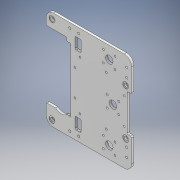
# Autodesk Inventor part: new_torso_topplate
Saved by Autodesk Inventor 2018 (Build 220112000, 112)
## iProperties
Created: 2017-02-16
Part Number: new_torso_topplate
Material: Aluminum 2014-T4
Document SubType Name: Modeling
Designer: steve
Mass: 92.2166 g
Surface Area: 250.436 cm^2
Volume: 32.9345 cm^3
Density: 2.8 g/cm^3
Appearance: Satin
torso_topplate_W: 133,000 mm
torso_topplate_l_to_fit: 82,000 mm
torso_topplate_d: 3,000 mm
fit_w: 85,000 mm
fit_d: 25,500 mm
torso_topplate_total_l: 110,000 mm
stock_6_width: 6,250 mm
pillar_block_length: 20,000 mm
pillar_block_width: 20,000 mm
pillar_width: 15,000 mm
stock_3_width: 3,000 mm
pillar_length: 80,000 mm
pillar_plate_length: 60,000 mm
cover_d: 3,500 mm
Author: steve
Autodesk Inventor part; units mm, degrees
ref_plane "YZ Plane" through (0, 0, 0) normal (1, 0, 0) x (0, 1, 0)
ref_plane "XZ Plane" through (0, 0, 0) normal (0, 1, 0) x (-1, 0, 0)
ref_plane "XY Plane" through (0, 0, 0) normal (0, 0, 1) x (1, 0, 0)
sketch "Sketch1" plane through (0, 0, 0) normal (0, 1, 0) x (-1, 0, 0)
  line L0 (-41, 66.5) -> (41, 66.5) construction
  line L1 (41, 66.5) -> (41, -66.5) construction
  line L2 (41, -66.5) -> (-41, -66.5) construction
  line L3 (-41, -66.5) -> (-41, 66.5) construction
  line L4 (-41, 66.5) -> (41, -66.5) construction
  line L5 (41, 66.5) -> (-41, -66.5) construction
  line L6 (106.5296, 0) -> (-65.5883, 0) construction
  line L7 (66.5, -42.5) -> (61.25, -42.5) construction
  line L8 (41, -42.5) -> (41, 42.5) construction
  line L9 (41, 42.5) -> (66.5, 42.5) construction
  line L10 (66.5, 42.5) -> (66.5, -42.5) construction
  line L11 (66.5, -42.5) -> (41, 42.5) construction
  line L12 (41, -42.5) -> (66.5, 42.5) construction
  line L13 (74, 66.5) -> (74, -66.5) construction
  line L14 (-41, 66.5) -> (74, 66.5)
  line L15 (74, 66.5) -> (74, -66.5)
  line L16 (74, -66.5) -> (-41, -66.5)
  line L17 (-41, -66.5) -> (-41, 66.5)
  circle A0 centre (65.4393, 41.4393) radius 1.5 construction
  line L18 (66.5, 42.5) -> (60.0868, 36.0868) construction
  line L19 (66.5, 42.5) -> (75.5696, 42.5) construction
  line L20 (66.5, -42.5) -> (64.7221, -40.7221) construction
  line L21 (66.5, -42.5) -> (69.0143, -42.5) construction
  line L22 (41, -42.5) -> (42.6048, -40.8952) construction
  line L23 (41, -42.5) -> (43.2695, -42.5) construction
  line L24 (41, 42.5) -> (46.0799, 37.4201) construction
  line L25 (41, 42.5) -> (48.184, 42.5) construction
  circle A1 centre (42.0607, 41.4393) radius 1.5 construction
  circle A2 centre (65.4393, -41.4393) radius 1.5 construction
  circle A3 centre (42.0607, -41.4393) radius 1.5 construction
  line L26 (43.1213, 42.5) -> (46.25, 42.5)
  line L27 (66.5, 40.3787) -> (66.5, -40.3787)
  line L28 (64.3787, -42.5) -> (61.25, -42.5)
  line L29 (41, -40.3787) -> (41, 40.3787)
  arc A4 (66.5, 40.3787) -> (64.3787, 42.5) centre (65.4393, 41.4393) ccw construction
  arc A5 (64.3787, -42.5) -> (66.5, -40.3787) centre (65.4393, -41.4393) ccw construction
  arc A6 (41, -40.3787) -> (43.1213, -42.5) centre (42.0607, -41.4393) ccw
  arc A7 (43.1213, 42.5) -> (41, 40.3787) centre (42.0607, 41.4393) ccw
  line L30 (81.9414, -45.5) -> (23.4915, -45.5) construction
  line L31 (53.75, 61.7827) -> (53.75, -107.6212) construction
  line L32 (46.25, -34.6173) -> (61.25, -34.6173) construction
  line L33 (61.25, -34.6173) -> (61.25, -50.3827) construction
  line L34 (61.25, -50.3827) -> (46.25, -50.3827) construction
  line L35 (46.25, -50.3827) -> (46.25, -34.6173) construction
  line L36 (46.25, -34.6173) -> (61.25, -50.3827) construction
  line L37 (61.25, -34.6173) -> (46.25, -50.3827) construction
  arc A8 (46.25, -42.5) -> (61.25, -42.5) centre (53.75, -34.625) ccw
  line L38 (61.25, -42.5) -> (41, -42.5) construction
  line L39 (61.25, -42.5) -> (46.25, -42.5) construction
  line L40 (46.25, -42.5) -> (43.1213, -42.5)
  arc A9 (61.25, 42.5) -> (46.25, 42.5) centre (53.75, 34.625) ccw
  line L41 (61.25, 42.5) -> (64.3787, 42.5)
  line L42 (46.25, 42.5) -> (61.25, 42.5) construction
  line L43 (64.3787, 42.5) -> (66.5, 42.5)
  line L44 (66.5, 42.5) -> (66.5, 40.3787)
  line L45 (64.3787, -42.5) -> (66.5, -42.5)
  line L46 (66.5, -42.5) -> (66.5, -40.3787)
  point P0 (0, 0)
  point P1 (53.75, 0)
  point P2 (53.75, 0)
  point P3 (53.75, -42.5)
  dimension "d0" = 133
  dimension "d1" = 82
  dimension "d2" = 25.5
  dimension "d3" = 85
  dimension "d4" = 7.5
  dimension "d6" = 3
  dimension "d7" = 135
  dimension "d8" = 135
  dimension "d9" = 45
  dimension "d10" = 45
  dimension "d11" = 3
  dimension "d12" = 3
  dimension "d13" = 3
  dimension "d99" = 15
  dimension "d100" = 3
  constraints: 92 end point, 24 point on circle, 17 point on line, 11 horizontal, 11 midpoint, 10 centre point, 9 parallel, 5 perpendicular, 4 coincident, 4 equal length, 3 collinear, 3 symmetric about line, 2 vertical, 1 tangent, 1 other
  measures "d0" distance of L0.end L1.end
  measures "d1" distance of L1.end L2.end
  measures "d2" distance of L7.start L8.start
  measures "d3" distance of L9.end L7.start
  measures "d4" distance between parallel lines of L13 L10
  measures "d6" diameter of A0
  measures "d7" angle of L18 L19
  measures "d8" angle of L21 L20
  measures "d9" angle of L23 L22
  measures "d10" angle of L24 L25
  measures "d11" diameter of A3
  measures "d12" diameter of A2
  measures "d13" diameter of A1
  measures "d99" distance of L33.end L34.end
  measures "d100" distance between parallel lines of L7 L30
extrude "Extrusion1" add sketch "Sketch1" along normal blind 3
fillet "Fillet1" radius 10 4 edges at (41, 1.5, 66.5) (41, 1.5, -66.5) (-74, 1.5, -66.5) (-74, 1.5, 66.5)
sketch "Sketch2" plane through (0, 3, 0) normal (0, 1, 0) x (1, 0, 0)
  arc A0 (-74, -56.5) -> (-64, -66.5) centre (-64, -56.5) ccw construction
  line L0 (-64, -66.5) -> (31, -66.5) construction
  arc A1 (31, -66.5) -> (41, -56.5) centre (31, -56.5) ccw construction
  line L1 (41, -56.5) -> (41, 56.5) construction
  arc A2 (41, 56.5) -> (31, 66.5) centre (31, 56.5) ccw construction
  line L2 (31, 66.5) -> (-64, 66.5) construction
  arc A3 (-64, 66.5) -> (-74, 56.5) centre (-64, 56.5) ccw construction
  line L3 (-74, 56.5) -> (-74, -56.5) construction
  line L4 (-66.5, -42.5) -> (-66.5, 42.5) construction
  line L5 (-66.5, 42.5) -> (-61.25, 42.5) construction
  arc A4 (-41, 40.3787) -> (-43.1213, 42.5) centre (-42.0607, 41.4393) ccw construction
  line L6 (-41, 40.3787) -> (-41, -40.3787) construction
  arc A5 (-43.1213, -42.5) -> (-41, -40.3787) centre (-42.0607, -41.4393) ccw construction
  line L7 (-43.1213, -42.5) -> (-46.25, -42.5) construction
  line L8 (31.25, -56.5) -> (37.5, -56.5) construction
  line L9 (37.5, -56.5) -> (37.5, -36.5) construction
  line L10 (37.5, -36.5) -> (31.25, -36.5) construction
  line L11 (31.25, -36.5) -> (31.25, -56.5) construction
  line L12 (37.5, 78) -> (37.5, -82) construction
  line L13 (41, -56.5) -> (-13.5, -56.5) construction
  line L14 (41, -56.5) -> (41, 56.5) construction
  line L15 (41, 56.5) -> (10.5, 56.5) construction
  line L16 (31.25, 36.5) -> (37.5, 36.5) construction
  line L17 (37.5, 36.5) -> (37.5, 56.5) construction
  line L18 (37.5, 56.5) -> (31.25, 56.5) construction
  line L19 (31.25, 56.5) -> (31.25, 36.5) construction
  line L20 (34.375, -36.5) -> (34.375, -56.5) construction
  line L21 (34.375, 36.5) -> (34.375, 56.5) construction
  line L22 (31.25, 46.5) -> (48, 46.5) construction
  line L23 (31.25, -46.5) -> (52, -46.5) construction
  line L24 (-75, -63) -> (42, -63) construction
  line L25 (-71, 63) -> (42, 63) construction
  line L26 (-46, -105.44) -> (-46, 104.2053) construction
  line L27 (-41, 40.3787) -> (-41, -40.3787) construction
  line L28 (-46, -63) -> (-26, -63) construction
  line L29 (-26, -63) -> (-26, -56.75) construction
  line L30 (-26, -56.75) -> (-46, -56.75) construction
  line L31 (-46, -56.75) -> (-46, -63) construction
  line L32 (-46, -59.875) -> (-26, -59.875) construction
  line L33 (-36, -56.75) -> (-36, -63) construction
  line L34 (-46, 56.75) -> (-26, 56.75) construction
  line L35 (-26, 56.75) -> (-26, 63) construction
  line L36 (-26, 63) -> (-46, 63) construction
  line L37 (-46, 63) -> (-46, 56.75) construction
  line L38 (-46, 59.875) -> (-26, 59.875) construction
  line L39 (-36, 63) -> (-36, 56.75) construction
  arc A6 (-61.25, -42.5) -> (-46.25, -42.5) centre (-53.75, -34.625) ccw projected
  line L40 (-61.25, -42.5) -> (-66.5, -42.5) projected
  arc A7 (-46.25, 42.5) -> (-61.25, 42.5) centre (-53.75, 34.625) ccw projected
  line L41 (-46.25, 42.5) -> (-43.1213, 42.5) projected
  point P0 (0, 0)
  point P1 (34.375, -52.5)
  point P2 (34.375, -40.5)
  point P3 (34.375, 40.5)
  point P4 (34.375, 52.5)
  point P5 (-30, 59.875)
  point P6 (-42, 59.875)
  point P7 (-30, -59.875)
  point P8 (-42, -59.875)
  dimension "d17" = 20
  dimension "d18" = 6.25
  dimension "d19" = 3.5
  dimension "d20" = 20
  dimension "d21" = 6.25
  dimension "d24" = 3.5
  dimension "d25" = 3.5
  dimension "d26" = 6.25
  dimension "d27" = 20
  dimension "d28" = 6.25
  dimension "d29" = 20
  dimension "d32" = 6
  dimension "d33" = 6
  dimension "d34" = 6
  dimension "d35" = 6
  dimension "d36" = 6
  dimension "d37" = 6
  dimension "d38" = 6
  dimension "d39" = 6
  dimension "d61" = 5
  constraints: 60 end point, 13 midpoint, 10 horizontal, 9 point on line, 8 collinear, 8 parallel, 5 perpendicular, 1 vertical
  measures "d17" distance of L10.end L8.start
  measures "d18" distance of L8.start L8.end
  measures "d19" distance between parallel lines of L1 L12
  measures "d20" distance of L18.end L19.end
  measures "d21" distance of L19.end L16.end
  measures "d24" distance between parallel lines of L0 L24
  measures "d25" distance between parallel lines of L2 L25
  measures "d26" distance of L28.end L29.end
  measures "d27" distance of L29.end L30.end
  measures "d28" distance of L34.end L36.start
  measures "d29" distance of L36.start L37.start
  measures "d32" distance from line of L33 point (-42, -59.875)
  measures "d33" distance from line of L33 point (-30, -59.875)
  measures "d34" distance from line of L23 point (34.375, -52.5)
  measures "d35" distance from line of L23 point (34.375, -40.5)
  measures "d36" distance from line of L22 point (34.375, 40.5)
  measures "d37" distance from line of L22 point (34.375, 52.5)
  measures "d38" distance from line of L39 point (-30, 59.875)
  measures "d39" distance from line of L39 point (-42, 59.875)
  measures "d61" distance between parallel lines of L27 L26
hole "Hole1" at (34.375, 3, 52.5) at (34.375, 3, 40.5) at (34.375, 3, -40.5) at (34.375, 3, -52.5) at (-30, 3, -59.875) at (-42, 3, -59.875) at (-30, 3, 59.875) at (-42, 3, 59.875) direction (0, -1, 0) diameter 3 end through all countersink diameter 4 countersink angle 90
sketch "Sketch4" plane through (0, 3, 0) normal (0, 1, 0) x (1, 0, 0)
  line L0 (11, -83) -> (11, 74) construction
  line L1 (41, -56.5) -> (41, 56.5) construction
  line L2 (-83, -50) -> (80, -50) construction
  line L3 (-64, -66.5) -> (31, -66.5) construction
  circle A0 centre (11, -50) radius 5
  line L4 (112.6, 0) -> (-115.6, 0) construction
  circle A1 centre (11, 50) radius 5
  point P0 (0, 0)
  dimension "d48" = 30
  dimension "d49" = 16.5
  dimension "d50" = 10
  constraints: 4 end point, 2 centre point, 2 point on line, 1 horizontal, 1 symmetric about line, 1 vertical, 1 other
  measures "d48" distance between parallel lines of L1 L0
  measures "d49" distance between parallel lines of L2 L3
  measures "d50" diameter of A0
extrude "Extrusion2" cut sketch "Sketch4" against normal blind 3
sketch "Sketch5" plane through (0, 3, 0) normal (0, 1, 0) x (1, 0, 0)
  circle A0 centre (11, -50) radius 11 construction
  circle A1 centre (11, -50) radius 5 construction
  line L0 (18.7782, -42.2218) -> (3.2218, -42.2218) construction
  line L1 (3.2218, -42.2218) -> (3.2218, -57.7782) construction
  line L2 (3.2218, -57.7782) -> (18.7782, -57.7782) construction
  line L3 (18.7782, -57.7782) -> (18.7782, -42.2218) construction
  line L4 (18.7782, -42.2218) -> (3.2218, -57.7782) construction
  line L5 (3.2218, -42.2218) -> (18.7782, -57.7782) construction
  line L6 (-97, 0) -> (64, 0) construction
  circle A2 centre (11, 50) radius 11 construction
  circle A3 centre (11, 50) radius 5 construction
  line L7 (18.7782, 42.2218) -> (3.2218, 42.2218) construction
  line L8 (3.2218, 42.2218) -> (3.2218, 57.7782) construction
  line L9 (3.2218, 57.7782) -> (18.7782, 57.7782) construction
  line L10 (18.7782, 57.7782) -> (18.7782, 42.2218) construction
  line L11 (18.7782, 42.2218) -> (3.2218, 57.7782) construction
  line L12 (3.2218, 42.2218) -> (18.7782, 57.7782) construction
  point P0 (0, 0)
  dimension "d53" = 22
  constraints: 24 end point, 10 symmetric about line, 8 coincident, 4 midpoint, 2 horizontal, 2 parallel, 2 perpendicular, 1 centre point, 8 other
hole "Hole2" at (3.2218, 3, 42.2218) at (18.7782, 3, 42.2218) at (18.7782, 3, 57.7782) at (3.2218, 3, 57.7782) at (3.2218, 3, -57.7782) at (18.7782, 3, -57.7782) at (18.7782, 3, -42.2218) at (3.2218, 3, -42.2218) direction (0, -1, 0) diameter 2.5 end through all
sketch "Sketch6" plane through (0, 3, 0) normal (0, 1, 0) x (1, 0, 0)
  line L0 (-97, 0) -> (64, 0) construction
  circle A0 centre (16, 0) radius 5
  circle A1 centre (16, 0) radius 11 construction
  line L1 (23.7782, 7.7782) -> (8.2218, 7.7782) construction
  line L2 (8.2218, 7.7782) -> (8.2218, -7.7782) construction
  line L3 (8.2218, -7.7782) -> (23.7782, -7.7782) construction
  line L4 (23.7782, -7.7782) -> (23.7782, 7.7782) construction
  line L5 (23.7782, 7.7782) -> (8.2218, -7.7782) construction
  line L6 (8.2218, 7.7782) -> (23.7782, -7.7782) construction
  circle A2 centre (8.2218, -7.7782) radius 1.25
  circle A3 centre (8.2218, 7.7782) radius 1.25
  circle A4 centre (23.7782, -7.7782) radius 1.25
  circle A5 centre (23.7782, 7.7782) radius 1.25
  line L7 (41, -56.5) -> (41, 56.5) projected
  point P0 (0, 0)
  dimension "d63" = 22
  dimension "d62" = 10
  dimension "d64" = 2.5
  dimension "d65" = 25
  constraints: 12 end point, 5 centre point, 4 coincident, 3 equal radius, 2 midpoint, 2 parallel, 2 perpendicular, 1 horizontal, 1 point on line, 4 other
  measures "d62" diameter of A0
  measures "d64" diameter of A2
  measures "d65" distance from line of L7 A0.centre
extrude "Extrusion3" cut sketch "Sketch6" against normal through all
sketch "Sketch7" plane through (0, 0, 0) normal (0, -1, 0) x (1, 0, 0)
  line L0 (41, 56.5) -> (41, -56.5) construction
  line L1 (41, 0) -> (-82.9368, 0) construction
  line L2 (35, -25) -> (41, -25)
  line L3 (41, -25) -> (41, 25)
  line L4 (41, 25) -> (35, 25)
  line L5 (35, 25) -> (35, -25)
  line L6 (35, -25) -> (41, 25) construction
  line L7 (41, -25) -> (35, 25) construction
  point P0 (0, 0)
  point P1 (38, 0)
  dimension "d68" = 6
  dimension "d69" = 50
  constraints: 14 end point, 3 midpoint, 2 horizontal, 2 parallel, 2 point on line, 1 perpendicular
  measures "d68" distance of L2.start L2.end
  measures "d69" distance of L4.end L2.start
extrude "Extrusion4" cut sketch "Sketch7" against normal through all
fillet "Fillet2" radius 1.5 4 edges at (35, 1.5, 25) (35, 1.5, -25) (41, 1.5, -25) (41, 1.5, 25)
sketch "Sketch8" plane through (0, 3, 0) normal (0, 1, 0) x (1, 0, 0)
  line L0 (31, -17.75) -> (-35, -17.75) construction
  line L1 (-35, -17.75) -> (-35, 17.75) construction
  line L2 (-35, 17.75) -> (31, 17.75) construction
  line L3 (31, 17.75) -> (31, -17.75) construction
  line L4 (31, -17.75) -> (-35, 17.75) construction
  line L5 (-35, -17.75) -> (31, 17.75) construction
  line L6 (64, 0) -> (-97, 0) construction
  line L7 (7.0558, -33) -> (-28.4442, -33) construction
  line L8 (-28.4442, -33) -> (-28.4442, 33) construction
  line L9 (-28.4442, 33) -> (7.0558, 33) construction
  line L10 (7.0558, 33) -> (7.0558, -33) construction
  line L11 (7.0558, -33) -> (-28.4442, 33) construction
  line L12 (-28.4442, -33) -> (7.0558, 33) construction
  line L13 (-41, 40.3787) -> (-41, -40.3787) projected
  point P0 (0, 0)
  point P1 (-2, 0)
  point P2 (-2, 0)
  point P3 (-10.6942, 0)
  dimension "d73" = 35.5
  dimension "d74" = 66
  dimension "d77" = 35.5
  dimension "d78" = 66
  dimension "d115" = 6
  constraints: 24 end point, 8 coincident, 5 midpoint, 4 parallel, 2 horizontal, 2 perpendicular, 2 point on line
  measures "d73" distance of L0.end L1.end
  measures "d74" distance of L1.end L2.end
  measures "d77" distance of L8.end L9.end
  measures "d78" distance of L7.end L8.end
  measures "d115" distance between parallel lines of L1 L13
hole "Hole3" at (-28.4442, 3, 33) at (7.0558, 3, 33) at (7.0558, 3, -33) at (-28.4442, 3, -33) at (-35, 3, -17.75) at (-35, 3, 17.75) at (31, 3, 17.75) at (31, 3, -17.75) direction (0, -1, 0) diameter 2.5 end through all
sketch "Sketch10" plane through (0, 0, 0) normal (0, -1, 0) x (1, 0, 0)
  line L0 (-81.0677, 46.5) -> (54.948, 46.5) construction
  line L1 (-31, 73.2043) -> (-31, -77.9028) construction
  line L2 (31, 66.5) -> (-64, 66.5) construction
  line L3 (-108.2708, 0) -> (82.1512, 0) construction
  line L4 (-41, 40.3787) -> (-41, -40.3787) projected
  line L5 (-28.5, 38.75) -> (-33.5, 38.75)
  line L6 (-35, 40.25) -> (-35, 52.75)
  line L7 (-33.5, 54.25) -> (-28.5, 54.25)
  line L8 (-27, 52.75) -> (-27, 40.25)
  line L9 (-27, 38.75) -> (-35, 54.25) construction
  line L10 (-35, 38.75) -> (-27, 54.25) construction
  arc A0 (-35, 40.25) -> (-33.5, 38.75) centre (-33.5, 40.25) ccw
  arc A1 (-33.5, 54.25) -> (-35, 52.75) centre (-33.5, 52.75) ccw
  arc A2 (-27, 52.75) -> (-28.5, 54.25) centre (-28.5, 52.75) ccw
  arc A3 (-28.5, 38.75) -> (-27, 40.25) centre (-28.5, 40.25) ccw
  line L11 (-28.5, -38.75) -> (-33.5, -38.75)
  line L12 (-35, -40.25) -> (-35, -52.75)
  line L13 (-33.5, -54.25) -> (-28.5, -54.25)
  line L14 (-27, -52.75) -> (-27, -40.25)
  arc A4 (-33.5, -38.75) -> (-35, -40.25) centre (-33.5, -40.25) ccw
  arc A5 (-35, -52.75) -> (-33.5, -54.25) centre (-33.5, -52.75) ccw
  arc A6 (-28.5, -54.25) -> (-27, -52.75) centre (-28.5, -52.75) ccw
  arc A7 (-27, -40.25) -> (-28.5, -38.75) centre (-28.5, -40.25) ccw
  point P0 (0, 0)
  point P1 (-31, 46.5)
  dimension "d92" = 20
  dimension "d95" = 10
  dimension "d96" = 15.5
  dimension "d97" = 8
  dimension "d98" = 1.5
  constraints: 24 end point, 16 point on circle, 12 symmetric about line, 10 point on line, 8 centre point, 8 tangent, 3 equal radius, 2 horizontal, 2 midpoint, 2 parallel, 1 perpendicular, 1 vertical, 4 other
  measures "d92" distance between parallel lines of L2 L0
  measures "d95" distance between parallel lines of L4 L1
  measures "d96" distance of L10.start L9.end
  measures "d97" distance of L9.end L10.end
  measures "d98" radius of A0
extrude "Extrusion6" cut sketch "Sketch10" against normal through all
sketch "Sketch11" plane through (0, 3, 0) normal (0, 1, 0) x (1, 0, 0)
  line L0 (38, -57.2977) -> (38, -10.4213) construction
  circle A0 centre (33, -31) radius 5 construction
  line L1 (35, -23.5) -> (35, 23.5) construction
  line L2 (-97, 0) -> (64, 0) construction
  line L3 (39.5, -25) -> (36.5, -25) construction
  line L4 (41, -56.5) -> (41, -26.5) construction
  circle A1 centre (-66, -58.5) radius 5 construction
  line L5 (-71, -65.8975) -> (-71, -94.3992) construction
  line L6 (-74, 56.5) -> (-74, -56.5) construction
  line L7 (-64, -66.5) -> (31, -66.5) construction
  circle A2 centre (33, 31) radius 5 construction
  circle A3 centre (-66, 58.5) radius 5 construction
  point P0 (0, 0)
  dimension "d101" = 10
  dimension "d103" = 6
  dimension "d104" = 3
  dimension "d105" = 10
  dimension "d106" = 3
  dimension "d107" = 8
  constraints: 4 centre point, 4 end point, 3 coincident, 3 symmetric about line, 2 tangent, 2 vertical, 2 other
  measures "d101" diameter of A0
  measures "d103" distance from line of L3 A0.centre
  measures "d104" distance between parallel lines of L0 L4
  measures "d105" diameter of A1
  measures "d106" distance between parallel lines of L6 L5
  measures "d107" distance from line of L7 A1.centre
hole "Hole4" at (-66, 3, 58.5) at (33, 3, 31) at (-66, 3, -58.5) at (33, 3, -31) direction (0, -1, 0) diameter 5 end through all
sketch "Sketch13" plane through (0, 3, 0) normal (0, 1, 0) x (1, 0, 0)
  line L0 (-74, -56.5) -> (-74, 56.5) projected
  line L1 (-66.5, -42.5) -> (-74, -42.5)
  line L2 (-74, -42.5) -> (-74, 42.5)
  line L3 (-74, 42.5) -> (-66.5, 42.5)
  line L4 (-66.5, 42.5) -> (-66.5, -42.5)
  line L5 (-66.5, 42.5) -> (-61.25, 42.5) projected
  point P0 (0, 0)
  constraints: 8 end point, 2 parallel, 1 collinear, 1 horizontal, 1 perpendicular, 1 point on line
extrude "Extrusion7" cut sketch "Sketch13" against normal through all
fillet "Fillet4" radius 1.5 2 edges at (-74, 1.5, 42.5) (-74, 1.5, -42.5)
sketch "Sketch14" plane through (0, 0, 0) normal (0, -1, 0) x (1, 0, 0)
  circle A0 centre (33, 31) radius 2.5 projected
  circle A1 centre (-66, 58.5) radius 2.5 projected
  circle A2 centre (-66, -58.5) radius 2.5 projected
  circle A3 centre (33, -31) radius 2.5 projected
  circle A4 centre (33, 31) radius 4.05
  circle A5 centre (-66, 58.5) radius 4.05
  circle A6 centre (33, -31) radius 4.05
  circle A7 centre (-66, -58.5) radius 4.05
  point P0 (0, 0)
  dimension "d119" = 8.1
  dimension "d120" = 8.1
  dimension "d121" = 8.1
  dimension "d122" = 8.1
  constraints: 4 centre point, 4 coincident
  measures "d119" diameter of A4
  measures "d120" diameter of A6
  measures "d121" diameter of A5
  measures "d122" diameter of A7
extrude "Extrusion8" cut sketch "Sketch14" against normal blind 0.5
sketch "Sketch15" plane through (0, 0, 0) normal (0, -1, 0) x (1, 0, 0)
  line L0 (-46.25, 42.5) -> (-74, 42.5)
  line L1 (-74, 42.5) -> (-74, 47.5)
  line L2 (-74, 47.5) -> (-46.25, 47.5)
  line L3 (-46.25, 47.5) -> (-46.25, 42.5)
  line L4 (-74, 56.5) -> (-74, 44) projected
  point P0 (0, 0)
  dimension "d129" = 5
  constraints: 8 end point, 2 parallel, 1 coincident, 1 collinear, 1 horizontal, 1 perpendicular
  measures "d129" distance of L2.end L0.start
extrude "Extrusion9" cut sketch "Sketch15" against normal through all
fillet "Fillet6" radius 1.5 3 edges at (-46.25, 1.5, 42.5) (-46.25, 1.5, 47.5) (-74, 1.5, 47.5)
fillet_without_effect "Fillet7"
equation "\"d0\" = torso_topplate_W"
equation "\"d1\" = torso_topplate_l_to_fit"
equation "\"d2\" = fit_d"
equation "\"d3\" = fit_w"
equation "\"d14\" = torso_topplate_d"
equation "\"d17\" = pillar_block_width"
equation "\"d18\" = stock_6_width"
equation "\"d19\" = cover_d"
equation "\"d20\" = d22"
equation "\"d21\" = d23"
equation "\"d24\" = cover_d"
equation "\"d25\" = cover_d"
equation "\"d26\" = stock_6_width"
equation "\"d27\" = pillar_block_width"
equation "\"d28\" = d30"
equation "\"d29\" = d31"
equation "\"d61\" = back_pillar_to_fit"
equation "\"d51\" = torso_topplate_d"
equation "\"d65\" = head_fix_dist"
equation "\"torso_topplate_W\" = 133"
equation "\"torso_topplate_l_to_fit\" = 82"
equation "\"torso_topplate_d\" = 3"
equation "\"fit_w\" = 85"
equation "\"fit_d\" = 25.5"
equation "\"torso_topplate_total_l\" = 110"
equation "\"cover_d\" = 3.5"
equation "\"back_pillar_to_fit\" = 5"
equation "\"head_fix_dist\" = 25"
equation "\"pillar_block_width\" = 20"
equation "\"stock_6_width\" = 6.25"
equation "\"d22\" = 20"
equation "\"d23\" = 6.25"
equation "\"d30\" = 6.25"
equation "\"d31\" = 20"
body "Solid1"
